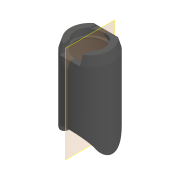
# Autodesk Inventor part: Socket
Saved by Autodesk Inventor 2020 (Build 240168000, 168)
## iProperties
Created: 2021-03-25
Part Number: Socket
Material: Generic
Document SubType Name: Modeling
Designer: deox
Density: 1 g/cm^3
Appearance: Generic
Author: deox
Autodesk Inventor part; units mm, degrees
ref_plane "YZ Plane" through (0, 0, 0) normal (1, 0, 0) x (0, 1, 0)
ref_plane "XZ Plane" through (0, 0, 0) normal (0, 1, 0) x (-1, 0, 0)
sketch "Sketch1" plane through (0, 0, 0) normal (0, 0, 1) x (1, 0, 0)
  line L0 (0, 0) -> (10.33, 0)
  line L1 (8.133, 28.571) -> (8.133, 26.271)
  line L2 (8.133, 26.271) -> (6.933, 26.271)
  line L3 (10.33, 0) -> (9.2116, 0)
  line L4 (0, 0) -> (0, 4.8929)
  line L5 (8.133, 28.571) -> (6.633, 28.571)
  line L6 (6.633, 28.571) -> (6.633, 30.501)
  line L7 (6.633, 30.501) -> (9.133, 30.501)
  line L8 (9.133, 30.501) -> (10.333, 30.501) construction
  line L9 (10.333, 30.501) -> (10.33, 26.501) construction
  line L10 (10.33, 26.501) -> (9.133, 30.501)
  line L11 (10.33, 26.501) -> (10.33, 0)
  line L12 (9.2116, 0) -> (9.2116, 24.534) construction
  line L13 (9.2116, 24.534) -> (10.33, 24.534)
  line L14 (10.33, 24.534) -> (8.88, 24.534)
  line L15 (8.88, 24.534) -> (8.5253, 24.534)
  line L16 (8.88, 24.534) -> (9.2116, 0)
  arc A0 (8.5253, 24.534) -> (6.933, 26.271) centre (4.9777, 22.8803) ccw
  line L17 (10.33, 0) -> (10.33, -10)
  line L18 (10.33, -10) -> (9.2116, -10)
  line L19 (9.2116, 0) -> (9.2116, -10)
  dimension "d0" = 10.33
  dimension "d10" = 2.3
  dimension "d11" = 1.2
  dimension "d12" = 1.1184
  dimension "d20" = 1.5
  dimension "d21" = 1.93
  dimension "d22" = 2.5
  dimension "d23" = 1.2
  dimension "d24" = 4
  dimension "d25" = 24.534
  dimension "d26" = 1.45
  dimension "d27" = 0.3547
  dimension "d46" = 10
  constraints: 40 end point, 7 perpendicular, 4 point on line, 3 horizontal, 3 vertical, 2 point on circle, 1 centre point
  measures "d0" distance of L0.end L0.start
  measures "d10" distance of L1.start L1.end
  measures "d11" distance of L1.end L2.end
  measures "d12" distance of L0.end L3.end
  measures "d20" distance of L1.start L5.end
  measures "d21" distance of L5.end L6.end
  measures "d22" distance of L6.end L7.end
  measures "d23" distance of L7.end L8.end
  measures "d24" distance of L8.end L9.end
  measures "d25" distance of L3.end L12.end
  measures "d26" distance of L13.end L14.end
  measures "d27" distance of L14.end L15.end
  measures "d46" distance of L0.end L17.end
revolve "Revolution1" add sketch "Sketch1" angle 360 about axis through (0, 0, 0) along (0, 1, 0)
sketch "Sketch2" plane through (0, 0, 0) normal (0, 0, 1) x (1, 0, 0)
  line L0 (-6.633, 30.501) -> (6.633, 30.501) projected
  line L1 (-9.133, 30.501) -> (9.133, 30.501) projected
  line L2 (0, 30.501) -> (-4.6, 30.501)
  line L3 (-4.6, 30.501) -> (-4.6, 26.511)
  line L4 (-4.6, 26.511) -> (0, 26.501)
  line L5 (-10.33, 26.501) -> (10.33, 26.501) projected
  line L6 (0, 30.501) -> (0, 31.8797)
  line L7 (0, 30.501) -> (4.6, 30.501)
  line L8 (4.6, 30.501) -> (4.6, 26.511)
  line L9 (4.6, 26.511) -> (0, 26.501)
  point P0 (0, 0)
  point P1 (4.6, 29.647)
  dimension "d28" = 4.6
  dimension "d29" = 3.99
  constraints: 14 end point, 2 midpoint, 2 symmetric about line, 1 perpendicular, 1 point on line, 1 vertical
  measures "d28" distance of L2.start L2.end
  measures "d29" distance of L2.end L3.end
extrude "Extrusion1" cut sketch "Sketch2" along normal blind 12.5
sketch "Sketch3" plane through (0, 0, 0) normal (1, 0, 0) x (0, 1, 0)
  line L0 (26.511, 6.7071) -> (26.511, 9.2459) projected
  line L1 (26.511, 9.2459) -> (27.3287, 8.9718)
  line L2 (26.511, 9.2459) -> (23.0647, 10.4013)
  line L3 (23.0647, 10.4013) -> (26.9199, 10.5302)
  line L4 (26.9199, 10.5302) -> (26.511, 9.2459)
  point P0 (0, 0)
  constraints: 8 end point, 1 point on line, 2 other
extrude "Extrusion2" cut sketch "Sketch3" against normal mid plane 12.5
sketch "Sketch4" plane through (0, 0, 0) normal (0, 0, 1) x (1, 0, 0)
  line L0 (-6.633, 30.501) -> (6.633, 30.501) projected
  line L1 (0, 30.501) -> (-4.6, 30.501)
  line L2 (-4.6, 30.501) -> (-4.6, 29.881)
  line L3 (-4.6, 30.501) -> (-4.6, 28.571) projected
  line L4 (-4.6, 29.881) -> (0, 29.881)
  line L5 (0, 30.501) -> (0, 31.4354)
  line L6 (0, 30.501) -> (4.6, 30.501)
  line L7 (4.6, 30.501) -> (4.6, 29.881)
  line L8 (4.6, 29.881) -> (0, 29.881)
  point P0 (0, 0)
  dimension "d32" = 4.6
  dimension "d33" = 0.62
  constraints: 14 end point, 1 collinear, 1 midpoint, 1 perpendicular, 1 point on line, 1 symmetric about line, 1 vertical
  measures "d32" distance of L1.start L1.end
  measures "d33" distance of L1.end L2.end
extrude "Extrusion3" cut sketch "Sketch4" against normal blind 12.5
sketch "Sketch5" plane through (0, 29.881, 0) normal (0, 1, 0) x (1, 0, 0)
  line L0 (0.256, 9.2303) -> (-0.256, 9.2303)
  line L1 (-0.256, 9.2303) -> (-0.256, 9.4068)
  line L2 (-0.256, 9.4068) -> (0.256, 9.4068)
  line L3 (0.256, 9.4068) -> (0.256, 9.2303)
  arc A0 (4.6, 8.104) -> (-4.6, 8.104) centre (0, 0) ccw projected
  line L4 (0.256, 9.2303) -> (-0.256, 9.4068) construction
  line L5 (-0.256, 9.2303) -> (0.256, 9.4068) construction
  point P0 (0, 9.3185)
  constraints: 12 end point, 2 midpoint, 2 parallel, 1 horizontal, 1 perpendicular, 1 point on circle
extrude "Extrusion4" cut sketch "Sketch5" against normal blind 0.01
ref_plane "Work Plane1" through (2.428, 29.881, -9.2303) normal (0, 0.9923319, -0.1236015) x (-1, 0, 0)
sketch "Sketch6" plane through (2.428, 29.881, -9.2303) normal (0, 0.9923319, -0.1236015) x (-1, 0, 0)
  line L0 (2.172, -0.0841) -> (2.172, 0) construction
  line L1 (2.172, 0) -> (2.684, 0) construction
  line L2 (2.684, 0) -> (2.684, -0.0841) construction
  ellipse E0 centre (2.428, 9.1595) end of major axis (-6.8905, 9.1595) minor radius 9.2471 (2.684, -0.0841) -> (7.028, 1.1177) ccw construction
  line L3 (7.028, 4.4174) -> (7.028, 1.1177) projected
  ellipse E1 centre (2.428, 9.1595) end of major axis (-4.205, 9.1595) minor radius 6.5821 (-2.172, 4.4174) -> (7.028, 4.4174) ccw construction
  line L4 (-2.172, 4.4174) -> (-2.172, 1.1177) projected
  ellipse E2 centre (2.428, 9.1595) end of major axis (-6.8905, 9.1595) minor radius 9.2471 (-2.172, 1.1177) -> (2.172, -0.0841) ccw construction
  ellipse E3 centre (2.428, 9.1595) end of major axis (-4.205, 9.1595) minor radius 6.5821 (-2.172, 4.4174) -> (7.028, 4.4174) ccw construction
  line L5 (-2.172, 4.4174) -> (-2.172, -1.9245)
  ellipse E4 centre (2.428, 8.9976) end of major axis (-5.705, 8.9976) minor radius 8.0706 (-2.172, 15.6533) -> (7.028, 15.6533) ccw construction
  line L6 (2.428, 8.9976) -> (2.428, -4.5406) construction
  ellipse E5 centre (2.428, 8.4986) end of major axis (-6.452, 8.4986) minor radius 8.8119 construction
  line L7 (-2.172, 4.4174) -> (-2.172, 1.1177) projected
  line L8 (-2.172, 4.4174) -> (2.428, 4.4174)
  line L9 (-2.172, -1.9245) -> (2.428, -1.9245)
  line L10 (7.028, 4.4174) -> (7.028, -1.9245)
  line L11 (7.028, 4.4174) -> (2.428, 4.4174)
  line L12 (7.028, -1.9245) -> (2.428, -1.9245)
  point P0 (2.428, 5.4662)
  point P1 (7.028, 1.1177)
  point P2 (-2.172, 1.1177)
  constraints: 14 end point, 2 horizontal, 2 point on line, 2 vertical, 1 symmetric about line, 6 other
extrude "Extrusion5" cut sketch "Sketch6" along normal blind 1.51 and the other way blind 0.551
sketch "Sketch7" plane through (0, 0, 0) normal (1, 0, 0) x (0, 1, 0)
  line L0 (28.571, -6.633) -> (29.6493, -6.633) projected
  line L1 (29.8802, -4.7788) -> (29.4475, -8.2529) projected
  line L2 (29.6493, -6.633) -> (29.5494, -7.4348)
  line L3 (29.2928, -9.4945) -> (26.501, -10.33) projected
  line L4 (26.501, -10.33) -> (27.868, -9.9209)
  arc A0 (29.5494, -7.4348) -> (27.868, -9.9209) centre (47.9732, -21.7066) ccw
  circle A1 centre (47.9732, -21.7066) radius 23.305
  line L5 (47.9732, 1.5984) -> (47.9732, -45.0115)
  point P0 (0, 0)
  dimension "d43" = 0.808
  dimension "d44" = 1.4269
  constraints: 6 end point, 5 point on circle, 2 centre point, 2 point on line, 1 coincident
  measures "d43" distance of L0.end L2.end
  measures "d44" distance of L3.end L4.end
revolve "Revolution2" cut sketch "Sketch7" angle 360 about axis through (0, 47.9732, 1.5984) along (0, 0, -1) contours A1 L5 A0
sketch "Sketch8" plane through (0, 0, 0) normal (0, 0, 1) x (1, 0, 0)
  line L0 (-9.2116, -10) -> (9.2116, -10) projected
  ellipse E0 centre (0, -10) end of major axis (9.2116, -10) minor radius 10
  point P0 (0, 0)
  constraints: 1 horizontal, 1 midpoint, 4 other
extrude "Extrusion6" cut sketch "Sketch8" against normal mid plane 46.75 contours E0 L0 picked at (3.0077, -8.8493)
sketch "Sketch9" plane through (0, 0, 0) normal (1, 0, 0) x (0, 1, 0)
  line L0 (-10, 4.675) -> (-10, -4.675) projected
  ellipse E0 centre (0, 0) end of major axis (-10, 0) minor radius 7.442 (-5.9841, 5.9624) -> (-5.9841, -5.9624) ccw
  line L1 (-5.9841, -5.9624) -> (-11.5111, -5.9624)
  line L2 (-11.5111, -5.9624) -> (-11.5111, 0)
  line L3 (-11.5111, 0) -> (-10.5603, 0)
  line L4 (-5.9841, 5.9624) -> (-11.5111, 5.9624)
  line L5 (-11.5111, 5.9624) -> (-11.5111, 0)
  constraints: 10 end point, 2 horizontal, 2 symmetric about line, 1 coincident, 1 perpendicular, 4 other
extrude "Extrusion7" cut sketch "Sketch9" against normal mid plane 46.75
sketch "Sketch10" plane through (0, 0, 0) normal (1, 0, 0) x (0, 1, 0)
  circle A0 centre (-5.5646, 0) radius 1.2
  point P0 (0, 0)
  dimension "d51" = 2.4
  constraints: 1 centre point
  measures "d51" diameter of A0
extrude "Extrusion8" add sketch "Sketch10" along normal blind 10 and the other way blind 10.125
sketch "Sketch11" plane through (0, 0, 0) normal (1, 0, 0) x (0, 1, 0)
  spline S0 degree 2 poles (-4.3646, 0) (-4.3646, -2.0785) (-6.1646, -1.0392) (-7.9646, 0) (-6.1646, 1.0392) (-4.3646, 2.0785) (-4.3646, 0) knots 0 0 0 0.333333 0.333333 0.666667 0.666667 1 1 1 weights 1 0.5 1 0.5 1 0.5 1 projected
  point P0 (0, 0)
  constraints: 1 other
extrude "Extrusion9" cut sketch "Sketch11" against normal mid plane 15.5
ref_plane "Work Plane2" through (0, -5.5646, 0) normal (1, 0, 0) x (0, 0, -1)
sketch "Sketch13" plane through (0, -5.5646, 0) normal (1, 0, 0) x (0, 0, -1)
  circle A0 centre (0, 0) radius 1.2 projected
  circle A1 centre (0, 0) radius 3
  point P0 (0, 5.5646)
  dimension "d61" = 6
  constraints: 1 centre point, 1 coincident
  measures "d61" diameter of A1
extrude "Extrusion11" cut sketch "Sketch13" against normal mid plane 18.5
body "Solid1"
